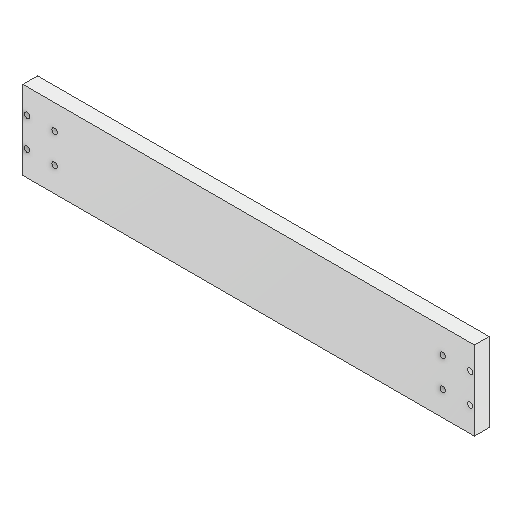
# Autodesk Inventor part: Part132
Saved by Autodesk Inventor 2026.2 (Build 302298000, 298)
## iProperties
Created: 2026-03-10
Part Number: Part132
Material: ABS Plastic
Document SubType Name: Modeling
Designer: gaoet
Density: 1.06 g/cm^3
Appearance: Smooth - White
Author: gaoet
Autodesk Inventor part; units mm, degrees
ref_plane "YZ Plane" through (0, 0, 0) normal (1, 0, 0) x (0, 1, 0)
ref_plane "XZ Plane" through (0, 0, 0) normal (0, 1, 0) x (-1, 0, 0)
ref_plane "XY Plane" through (0, 0, 0) normal (0, 0, 1) x (1, 0, 0)
sketch "Sketch1" plane through (0, 0, 0) normal (0, 0, 1) x (1, 0, 0)
  line L0 (-123, 21.5) -> (123, 21.5)
  line L1 (123, 21.5) -> (123, -21.5)
  line L2 (123, -21.5) -> (-123, -21.5)
  line L3 (-123, -21.5) -> (-123, 21.5)
  line L4 (-123, 21.5) -> (123, -21.5) construction
  line L5 (123, 21.5) -> (-123, -21.5) construction
  line L6 (0, -155.5635) -> (155.5635, 0) construction
  line L7 (155.5635, 0) -> (0, 155.5635) construction
  line L8 (0, 155.5635) -> (-155.5635, 0) construction
  line L9 (-155.5635, 0) -> (0, -155.5635) construction
  line L10 (0, -155.5635) -> (0, 155.5635) construction
  line L11 (155.5635, 0) -> (-155.5635, 0) construction
  line L12 (0, -155.5635) -> (220, -155.5635) construction
  line L13 (-120.75, -8) -> (120.75, -8)
  line L14 (120.75, -8) -> (120.75, 8)
  line L15 (120.75, 8) -> (-120.75, 8)
  line L16 (-120.75, 8) -> (-120.75, -8)
  line L17 (-120.75, -8) -> (120.75, 8) construction
  line L18 (120.75, -8) -> (-120.75, 8) construction
  line L19 (-105.75, -8) -> (105.75, -8)
  line L20 (105.75, -8) -> (105.75, 8)
  line L21 (105.75, 8) -> (-105.75, 8)
  line L22 (-105.75, 8) -> (-105.75, -8)
  line L23 (-105.75, -8) -> (105.75, 8) construction
  line L24 (105.75, -8) -> (-105.75, 8) construction
  point P0 (0, 0)
  dimension "d0" = 246
  dimension "d1" = 220
  dimension "d2" = 45
  dimension "d3" = 220
  dimension "d4" = 43
  dimension "d5" = 241.5
  dimension "d6" = 16
  dimension "d7" = 15
  constraints: 50 end point, 8 midpoint, 8 parallel, 4 horizontal, 4 perpendicular, 1 equal length, 1 point on line
  measures "d0" distance of L1.end L2.end
  measures "d1" distance of L6.start L6.end
  measures "d2" angle of L12 L6
  measures "d3" distance of L7.end L6.end
  measures "d4" distance of L2.end L0.start
  measures "d5" distance of L15.end L14.end
  measures "d6" distance of L14.end L13.end
  measures "d7" distance between parallel lines of L14 L20
extrude "Extrusion1" add sketch "Sketch1" along normal blind 8 contours L0 L1 L2 L3 | L16 L15 L22 L13 | L22 L15 L20 L13 | L20 L15 L14 L13
hole "Hole1" at (-105.75, -8, 0) at (-120.75, -8, 0) at (-120.75, 8, 0) at (-105.75, 8, 0) at (120.75, -8, 0) at (105.75, -8, 0) at (105.75, 8, 0) at (120.75, 8, 0) direction (0, 0, 1) diameter 3 end through all
body "Solid1"
